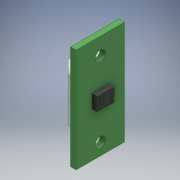
# Autodesk Inventor part: encoder
Saved by Autodesk Inventor 2018.3 (Build 223284000, 284)
## iProperties
Created: 2019-09-29
Part Number: encoder
Material: 一般
Document SubType Name: Modeling
Designer: Eiji Nishizawa
Density: 1 g/cm^3
Appearance: 滑らか - 濃い深緑
Author: Eiji Nishizawa
Autodesk Inventor part; units mm, degrees
ref_plane "YZ Plane" through (0, 0, 0) normal (1, 0, 0) x (0, 1, 0)
ref_plane "XZ Plane" through (0, 0, 0) normal (0, 1, 0) x (-1, 0, 0)
ref_plane "XY Plane" through (0, 0, 0) normal (0, 0, 1) x (1, 0, 0)
sketch "スケッチ1" plane through (0, 0, 0) normal (1, 0, 0) x (0, 1, 0)
  line L0 (7, 15) -> (-7, 15)
  line L1 (-7, 15) -> (-7, -15)
  line L2 (-7, -15) -> (7, -15)
  line L3 (7, -15) -> (7, 15)
  circle A0 centre (0, 10.05) radius 1.5
  circle A1 centre (0, -11.55) radius 1.5
  point P0 (0, 0)
  dimension "d0" = 14
  dimension "d1" = 30
  dimension "d2" = 7
  dimension "d3" = 15
  dimension "d4" = 3
  dimension "d5" = 3
  dimension "d6" = 3.45
  dimension "d7" = 3.45
  constraints: 8 end point, 2 centre point, 2 parallel, 1 horizontal, 1 perpendicular
  measures "d0" distance between parallel lines of L1 L3
  measures "d1" distance between parallel lines of L2 L0
  measures "d2" distance from line of L1 point (0, 0)
  measures "d3" distance from line of point (0, 0) L0
  measures "d4" diameter of A0
  measures "d5" diameter of A1
  measures "d6" distance edge to line of A0 L0
  measures "d7" distance from line of L2 A1.centre
extrude "押し出し1" add sketch "スケッチ1" along normal blind 1.6
sketch "スケッチ2" plane through (1.6, 0, 0) normal (1, 0, 0) x (0, 0, -1)
  line L0 (-2, 2.5) -> (2, 2.5)
  line L1 (2, 2.5) -> (2, -2.5)
  line L2 (2, -2.5) -> (-2, -2.5)
  line L3 (-2, -2.5) -> (-2, 2.5)
  point P0 (0, 0)
  dimension "d10" = 4
  dimension "d11" = 5
  dimension "d12" = 2.5
  dimension "d13" = 2
  constraints: 8 end point, 2 parallel, 1 horizontal, 1 perpendicular
  measures "d10" distance between parallel lines of L1 L3
  measures "d11" distance between parallel lines of L2 L0
  measures "d12" distance from line of L2 point (0, 0)
  measures "d13" distance from line of point (0, 0) L3
extrude "押し出し2" add sketch "スケッチ2" along normal blind 1.6
sketch "スケッチ3" plane through (0, 0, 0) normal (-1, 0, 0) x (0, 0, 1)
  line L0 (6.25, -5.725) -> (-6.25, -5.725)
  line L1 (-6.25, -5.725) -> (-6.25, 5.725)
  line L2 (-6.25, 5.725) -> (6.25, 5.725)
  line L3 (6.25, 5.725) -> (6.25, -5.725)
  line L4 (-15, -7) -> (-15, 7) projected
  line L5 (15, 7) -> (15, -7) projected
  point P0 (0, 0)
  dimension "d16" = 12.5
  dimension "d17" = 8.75
  dimension "d18" = 8.75
  dimension "d19" = 11.45
  dimension "d20" = 5.725
  dimension "d21" = 5.725
  constraints: 8 end point, 2 parallel, 1 horizontal, 1 perpendicular
  measures "d16" distance of L0.start L0.end
  measures "d17" distance between parallel lines of L4 L1
  measures "d18" distance between parallel lines of L5 L3
  measures "d19" distance of L2.end L0.start
  measures "d20" distance from line of point (0, 0) L2
  measures "d21" distance from line of point (0, 0) L0
extrude "押し出し3" add sketch "スケッチ3" along normal blind 6
chamfer "面取り1" distance 4 angle 45 1 edges at (-6, -5.725, 0)
